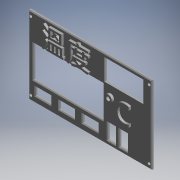
# Autodesk Inventor part: 溫度
Saved by Autodesk Inventor 2021 (Build 250183000, 183)
## iProperties
Part Number: 溫度
Material: 一般
Document SubType Name: 塑型
Designer: aura0
Appearance: 預設
Author: aura0
Autodesk Inventor part; units mm, degrees
ref_plane "YZ 平面" through (0, 0, 0) normal (1, 0, 0) x (0, 1, 0)
ref_plane "XZ 平面" through (0, 0, 0) normal (0, 1, 0) x (-1, 0, 0)
ref_plane "XY 平面" through (0, 0, 0) normal (0, 0, 1) x (1, 0, 0)
sketch "草圖1" plane through (0, 0, 0) normal (0, 0, 1) x (1, 0, 0)
  line L0 (-81, -51) -> (81, -51)
  line L1 (81, -51) -> (81, 51)
  line L2 (81, 51) -> (-81, 51)
  line L3 (-81, 51) -> (-81, -51)
  line L4 (-81, -51) -> (81, 51) construction
  line L5 (81, -51) -> (-81, 51) construction
  point P0 (0, 0)
  dimension "d0" = 162
  dimension "d1" = 102
  constraints: 12 end point, 2 midpoint, 2 parallel, 1 horizontal, 1 perpendicular
  measures "d0" distance of L2.end L1.end
  measures "d1" distance of L1.end L0.end
extrude "擠出1" add sketch "草圖1" along normal blind 3
sketch "草圖2" plane through (0, 0, 3) normal (0, 0, 1) x (1, 0, 0)
  line L0 (-75, -26) -> (17, -26)
  line L1 (17, -26) -> (17, 16)
  line L2 (17, 16) -> (-75, 16)
  line L3 (-75, 16) -> (-75, -26)
  line L4 (19, 19) -> (70, 19)
  line L5 (70, 19) -> (70, 47)
  line L6 (70, 47) -> (19, 47)
  line L7 (19, 47) -> (19, 19)
  line L8 (-72.2, -43) -> (-51.7, -43)
  line L9 (-51.7, -43) -> (-51.7, -32.5)
  line L10 (-51.7, -32.5) -> (-72.2, -32.5)
  line L11 (-72.2, -32.5) -> (-72.2, -43)
  line L12 (-41.2, -43) -> (-20.7, -43)
  line L13 (-20.7, -43) -> (-20.7, -32.5)
  line L14 (-20.7, -32.5) -> (-41.2, -32.5)
  line L15 (-41.2, -32.5) -> (-41.2, -43)
  line L16 (-10.2, -43) -> (10.3, -43)
  line L17 (10.3, -43) -> (10.3, -32.5)
  line L18 (10.3, -32.5) -> (-10.2, -32.5)
  line L19 (-10.2, -32.5) -> (-10.2, -43)
  line L20 (22.8, -45.9) -> (33.3, -45.9)
  line L21 (33.3, -45.9) -> (33.3, -25.4)
  line L22 (33.3, -25.4) -> (22.8, -25.4)
  line L23 (22.8, -25.4) -> (22.8, -45.9)
  line L24 (38.3, -45.9) -> (48.8, -45.9)
  line L25 (48.8, -45.9) -> (48.8, -25.4)
  line L26 (48.8, -25.4) -> (38.3, -25.4)
  line L27 (38.3, -25.4) -> (38.3, -45.9)
  line L28 (-81, -51) -> (81, -51) projected
  line L29 (-81, 51) -> (-81, -51) projected
  point P0 (0, 0)
  dimension "d4" = 8
  dimension "d5" = 8.8
  dimension "d6" = 10.5
  dimension "d7" = 10.5
  dimension "d8" = 10.5
  dimension "d9" = 20.5
  dimension "d10" = 20.5
  dimension "d11" = 20.5
  dimension "d12" = 10.5
  dimension "d13" = 25
  dimension "d14" = 6
  dimension "d15" = 92
  dimension "d16" = 42
  dimension "d17" = 5.1
  dimension "d18" = 10.5
  dimension "d19" = 10.5
  dimension "d20" = 20.5
  dimension "d21" = 5
  dimension "d22" = 103.8
  dimension "d23" = 70
  dimension "d24" = 100
  dimension "d25" = 51
  dimension "d26" = 28
  constraints: 56 end point, 14 parallel, 7 horizontal, 7 perpendicular, 6 point on line
  measures "d4" distance between parallel lines of L28 L8
  measures "d5" distance between parallel lines of L29 L11
  measures "d6" distance between parallel lines of L15 L9
  measures "d7" distance between parallel lines of L19 L13
  measures "d8" distance of L10.end L8.start
  measures "d9" distance of L8.start L8.end
  measures "d10" distance of L16.start L16.end
  measures "d11" distance of L12.start L12.end
  measures "d12" distance of L14.end L12.start
  measures "d13" distance between parallel lines of L28 L0
  measures "d14" distance between parallel lines of L29 L3
  measures "d15" distance of L0.start L0.end
  measures "d16" distance of L2.end L0.start
  measures "d17" distance between parallel lines of L28 L20
  measures "d18" distance of L24.start L24.end
  measures "d19" distance of L20.start L20.end
  measures "d20" distance of L22.end L20.start
  measures "d21" distance between parallel lines of L27 L21
  measures "d22" distance between parallel lines of L29 L23
  measures "d23" distance between parallel lines of L28 L4
  measures "d24" distance between parallel lines of L29 L7
  measures "d25" distance of L4.start L4.end
  measures "d26" distance of L4.end L5.end
extrude "擠出2" cut sketch "草圖2" against normal blind 3
sketch "草圖3" plane through (0, 0, 3) normal (0, 0, 1) x (1, 0, 0)
  line L0 (-63.5264, 47.7672) -> (2.568, 47.7672) construction
  line L1 (2.568, 47.7672) -> (2.568, 18.4539) construction
  line L2 (2.568, 18.4539) -> (-63.5264, 18.4539) construction
  line L3 (-63.5264, 18.4539) -> (-63.5264, 47.7672) construction
  line L4 (20.0661, 9.7884) -> (55.7099, 9.7884) construction
  line L5 (55.7099, 9.7884) -> (55.7099, -16.0486) construction
  line L6 (55.7099, -16.0486) -> (20.0661, -16.0486) construction
  line L7 (20.0661, -16.0486) -> (20.0661, 9.7884) construction
  line L8 (-32.3891, 19.2693) -> (-54.4492, 19.2693)
  line L9 (-54.4492, 19.2693) -> (-54.4492, 21.9303)
  line L10 (-54.4492, 21.9303) -> (-52.5822, 21.9303)
  line L11 (-52.5822, 21.9303) -> (-52.5822, 31.6727)
  line L12 (-52.5822, 31.6727) -> (-33.9771, 31.6727)
  line L13 (-33.9771, 31.6727) -> (-33.9771, 21.9303)
  line L14 (-33.9771, 21.9303) -> (-32.3891, 21.9303)
  line L15 (-32.3891, 21.9303) -> (-32.3891, 19.2693)
  line L16 (-34.6638, 33.7972) -> (-51.9813, 33.7972)
  line L17 (-51.9813, 33.7972) -> (-51.9813, 47.0805)
  line L18 (-51.9813, 47.0805) -> (-34.6638, 47.0805)
  line L19 (-34.6638, 47.0805) -> (-34.6638, 33.7972)
  line L20 (-37.5822, 36.4367) -> (-37.5822, 44.441)
  line L21 (-37.5822, 44.441) -> (-49.0414, 44.441)
  line L22 (-49.0414, 44.441) -> (-49.0414, 36.4367)
  line L23 (-49.0414, 36.4367) -> (-37.5822, 36.4367)
  spline S0 degree 2 poles (-53.7839, 29.2049) (-55.7367, 23.2393) (-58.6122, 18.4539) knots 0 0 0 1 1 1
  line L24 (-58.6122, 18.4539) -> (-61.0371, 20.3852)
  spline S1 degree 2 poles (-61.0371, 20.3852) (-58.2904, 25.0633) (-56.123, 31.029) knots 0 0 0 1 1 1
  line L25 (-56.123, 31.029) -> (-53.7839, 29.2049)
  line L26 (-38.0114, 38.9903) -> (-39.7281, 36.9303)
  spline S2 degree 2 poles (-39.7281, 36.9303) (-41.5092, 38.6255) (-43.505, 39.8058) knots 0 0 0 1 1 1
  spline S3 degree 2 poles (-43.505, 39.8058) (-45.1573, 38.0676) (-46.6809, 37.1878) knots 0 0 0 1 1 1
  line L27 (-46.6809, 37.1878) -> (-48.6122, 39.0547)
  spline S4 degree 2 poles (-48.6122, 39.0547) (-45.2217, 41.0075) (-43.9985, 43.9045) knots 0 0 0 1 1 1
  line L28 (-43.9985, 43.9045) -> (-41.2947, 43.5397)
  spline S5 degree 2 poles (-41.2947, 43.5397) (-41.4449, 42.6813) (-41.9813, 41.8444) knots 0 0 0 1 1 1
  spline S6 degree 2 poles (-41.9813, 41.8444) (-39.4921, 40.3423) (-38.0114, 38.9903) knots 0 0 0 1 1 1
  line L29 (-52.7539, 42.9388) -> (-54.8354, 40.6642)
  spline S7 degree 2 poles (-54.8354, 40.6642) (-56.7238, 42.8745) (-60.565, 45.4925) knots 0 0 0 1 1 1
  line L30 (-60.565, 45.4925) -> (-58.4835, 47.7028)
  spline S8 degree 2 poles (-58.4835, 47.7028) (-54.9427, 45.4066) (-52.7539, 42.9388) knots 0 0 0 1 1 1
  line L31 (-53.6552, 34.9775) -> (-55.5221, 32.6813)
  spline S9 degree 2 poles (-55.5221, 32.6813) (-57.7968, 35.0204) (-61.4663, 37.3594) knots 0 0 0 1 1 1
  line L32 (-61.4663, 37.3594) -> (-59.5994, 39.6985)
  spline S10 degree 2 poles (-59.5994, 39.6985) (-55.8226, 37.3165) (-53.6552, 34.9775) knots 0 0 0 1 1 1
  line L33 (-36.6595, 21.9303) -> (-36.6595, 29.0333)
  line L34 (-36.6595, 29.0333) -> (-39.2775, 29.0333)
  line L35 (-39.2775, 29.0333) -> (-39.2775, 21.9303)
  line L36 (-39.2775, 21.9303) -> (-36.6595, 21.9303)
  line L37 (-42.0243, 21.9303) -> (-42.0243, 29.0333)
  line L38 (-42.0243, 29.0333) -> (-44.5565, 29.0333)
  line L39 (-44.5565, 29.0333) -> (-44.5565, 21.9303)
  line L40 (-44.5565, 21.9303) -> (-42.0243, 21.9303)
  line L41 (-47.2603, 21.9303) -> (-47.2603, 29.0333)
  line L42 (-47.2603, 29.0333) -> (-49.771, 29.0333)
  line L43 (-49.771, 29.0333) -> (-49.771, 21.9303)
  line L44 (-49.771, 21.9303) -> (-47.2603, 21.9303)
  line L45 (0.744, 21.4367) -> (-0.1359, 18.6255)
  spline S11 degree 2 poles (-0.1359, 18.6255) (-6.0586, 18.9689) (-11.2732, 21.0933) knots 0 0 0 1 1 1
  spline S12 degree 2 poles (-11.2732, 21.0933) (-15.5436, 19.3122) (-21.4019, 18.5612) knots 0 0 0 1 1 1
  line L46 (-21.4019, 18.5612) -> (-22.7539, 21.3509)
  spline S13 degree 2 poles (-22.7539, 21.3509) (-17.6895, 21.6298) (-14.4921, 22.853) knots 0 0 0 1 1 1
  spline S14 degree 2 poles (-14.4921, 22.853) (-17.3676, 24.6556) (-18.9127, 27.7457) knots 0 0 0 1 1 1
  line L47 (-18.9127, 27.7457) -> (-20.3719, 27.7457)
  line L48 (-20.3719, 27.7457) -> (-20.3719, 30.3637)
  line L49 (-20.3719, 30.3637) -> (-3.0114, 30.3637)
  line L50 (-3.0114, 30.3637) -> (-3.0114, 27.7457)
  spline S15 degree 2 poles (-3.0114, 27.7457) (-4.7281, 25.1062) (-8.1401, 22.853) knots 0 0 0 1 1 1
  spline S16 degree 2 poles (-8.1401, 22.853) (-4.3848, 21.544) (0.744, 21.4367) knots 0 0 0 1 1 1
  line L51 (0.5508, 42.7457) -> (-22.4749, 42.7457)
  line L52 (-22.4749, 42.7457) -> (-22.4749, 31.9088)
  spline S17 degree 2 poles (-22.4749, 31.9088) (-22.4749, 23.7972) (-25.8869, 18.5612) knots 0 0 0 1 1 1
  line L53 (-25.8869, 18.5612) -> (-28.3547, 20.2135)
  spline S18 degree 2 poles (-28.3547, 20.2135) (-25.4363, 24.677) (-25.4363, 31.9088) knots 0 0 0 1 1 1
  line L54 (-25.4363, 31.9088) -> (-25.4363, 45.3637)
  line L55 (-25.4363, 45.3637) -> (-14.5779, 45.3637)
  spline S19 degree 2 poles (-14.5779, 45.3637) (-15.2217, 46.3509) (-15.844, 47.0805) knots 0 0 0 1 1 1
  line L56 (-15.844, 47.0805) -> (-12.6251, 47.7672)
  spline S20 degree 2 poles (-12.6251, 47.7672) (-11.9813, 46.6727) (-11.2517, 45.3637) knots 0 0 0 1 1 1
  line L57 (-11.2517, 45.3637) -> (0.5508, 45.3637)
  line L58 (0.5508, 45.3637) -> (0.5508, 42.7457)
  line L59 (0.229, 37.1019) -> (-4.6208, 37.1019)
  line L60 (-4.6208, 37.1019) -> (-4.6208, 32.2307)
  line L61 (-4.6208, 32.2307) -> (-17.3891, 32.2307)
  line L62 (-17.3891, 32.2307) -> (-17.3891, 37.1019)
  line L63 (-17.3891, 37.1019) -> (-21.359, 37.1019)
  line L64 (-21.359, 37.1019) -> (-21.359, 39.677)
  line L65 (-21.359, 39.677) -> (-17.3891, 39.677)
  line L66 (-17.3891, 39.677) -> (-17.3891, 41.6298)
  line L67 (-17.3891, 41.6298) -> (-14.5565, 41.6298)
  line L68 (-14.5565, 41.6298) -> (-14.5565, 39.677)
  line L69 (-14.5565, 39.677) -> (-7.5178, 39.677)
  line L70 (-7.5178, 39.677) -> (-7.5178, 41.6298)
  line L71 (-7.5178, 41.6298) -> (-4.6208, 41.6298)
  line L72 (-4.6208, 41.6298) -> (-4.6208, 39.677)
  line L73 (-4.6208, 39.677) -> (0.229, 39.677)
  line L74 (0.229, 39.677) -> (0.229, 37.1019)
  line L75 (-6.7668, 27.7457) -> (-15.5007, 27.7457)
  spline S21 degree 2 poles (-15.5007, 27.7457) (-14.1702, 25.7071) (-11.4019, 24.0976) knots 0 0 0 1 1 1
  spline S22 degree 2 poles (-11.4019, 24.0976) (-8.2689, 25.9002) (-6.7668, 27.7457) knots 0 0 0 1 1 1
  line L76 (-7.5178, 34.7843) -> (-7.5178, 37.1019)
  line L77 (-7.5178, 37.1019) -> (-14.5565, 37.1019)
  line L78 (-14.5565, 37.1019) -> (-14.5565, 34.7843)
  line L79 (-14.5565, 34.7843) -> (-7.5178, 34.7843)
  spline S23 degree 2 poles (26.8687, 9.7884) (28.8859, 9.7884) (31.7399, 6.9343) (31.7399, 4.96) knots 0 0 0 1 2 2 2
  spline S24 degree 2 poles (31.7399, 4.96) (31.7399, 2.9643) (28.8644, 0.0888) (26.8687, 0.0888) knots 0 0 0 1 2 2 2
  spline S25 degree 2 poles (26.8687, 0.0888) (24.8515, 0.0888) (21.9975, 2.9643) (21.9975, 4.96) knots 0 0 0 1 2 2 2
  spline S26 degree 2 poles (21.9975, 4.96) (21.9975, 6.9343) (24.873, 9.7884) (26.8687, 9.7884) knots 0 0 0 1 2 2 2
  spline S27 degree 2 poles (26.8687, 2.3635) (27.9417, 2.3635) (29.4438, 3.9085) (29.4438, 4.96) knots 0 0 0 1 2 2 2
  spline S28 degree 2 poles (29.4438, 4.96) (29.4438, 6.0115) (27.9417, 7.5137) (26.8687, 7.5137) knots 0 0 0 1 2 2 2
  spline S29 degree 2 poles (26.8687, 7.5137) (25.8172, 7.5137) (24.3151, 6.0115) (24.3151, 4.96) knots 0 0 0 1 2 2 2
  spline S30 degree 2 poles (24.3151, 4.96) (24.3151, 3.9085) (25.8172, 2.3635) (26.8687, 2.3635) knots 0 0 0 1 2 2 2
  spline S31 degree 2 poles (54.0146, -14.6322) (51.2464, -16.0486) (47.0404, -16.0486) knots 0 0 0 1 1 1
  spline S32 degree 2 poles (47.0404, -16.0486) (41.6112, -16.0486) (35.0876, -9.2031) (35.0876, -3.6237) knots 0 0 0 1 2 2 2
  spline S33 degree 2 poles (35.0876, -3.6237) (35.0876, 2.2347) (42.3193, 9.7884) (48.049, 9.7884) knots 0 0 0 1 2 2 2
  spline S34 degree 2 poles (48.049, 9.7884) (51.6326, 9.7884) (54.0146, 8.8012) knots 0 0 0 1 1 1
  line L80 (54.0146, 8.8012) -> (54.0146, 4.8742)
  spline S35 degree 2 poles (54.0146, 4.8742) (51.3751, 6.3549) (48.1777, 6.3549) knots 0 0 0 1 1 1
  spline S36 degree 2 poles (48.1777, 6.3549) (44.079, 6.3549) (39.1434, 0.9901) (39.1434, -3.3662) knots 0 0 0 1 2 2 2
  spline S37 degree 2 poles (39.1434, -3.3662) (39.1434, -7.5078) (43.7786, -12.6365) (47.6627, -12.6365) knots 0 0 0 1 2 2 2
  spline S38 degree 2 poles (47.6627, -12.6365) (51.2893, -12.6365) (54.0146, -10.9627) knots 0 0 0 1 1 1
  line L81 (54.0146, -10.9627) -> (54.0146, -14.6322)
  point P0 (0, 0)
  constraints: 4 other
extrude "擠出3" add sketch "草圖3" along normal blind 3
sketch "草圖4" plane through (0, 0, 3) normal (0, 0, 1) x (1, 0, 0)
  circle A0 centre (-77.9, 45) radius 1.8
  circle A1 centre (-77.9, -45) radius 1.8
  circle A2 centre (77.7, -45) radius 1.8
  circle A3 centre (77.7, 45) radius 1.8
  line L0 (-81, -51) -> (81, -51) projected
  line L1 (-81, 51) -> (-81, -51) projected
  point P0 (0, 0)
  dimension "d31" = 6
  dimension "d32" = 3.1
  dimension "d33" = 3.1
  dimension "d34" = 6
  dimension "d35" = 158.7
  dimension "d36" = 96
  dimension "d37" = 96
  dimension "d38" = 158.7
  dimension "d39" = 3.6
  dimension "d40" = 3.6
  dimension "d41" = 3.6
  dimension "d42" = 3.6
  constraints: 4 centre point
  measures "d31" distance from line of L0 A1.centre
  measures "d32" distance from line of L1 A1.centre
  measures "d33" distance from line of L1 A0.centre
  measures "d34" distance from line of L0 A2.centre
  measures "d35" distance from line of L1 A2.centre
  measures "d36" distance from line of L0 A0.centre
  measures "d37" distance from line of L0 A3.centre
  measures "d38" distance from line of L1 A3.centre
  measures "d39" diameter of A1
  measures "d40" diameter of A0
  measures "d41" diameter of A3
  measures "d42" diameter of A2
extrude "擠出4" cut sketch "草圖4" against normal blind 3
chamfer "倒角1" distance 1 angle 45 28 edges at (-29, 16, 3) (-29, -26, 3) (17, -5, 3) (-75, -5, 3) (-81, 0, 3) (0, 51, 3) (81, 0, 3) (0, -51, 3) (33.3, -35.65, 3) (28.05, -25.4, 3) (22.8, -35.65, 3) (28.05, -45.9, 3) (38.3, -35.65, 3) (43.55, -25.4, 3) (48.8, -35.65, 3) (43.55, -45.9, 3) (0.05, -43, 3) (10.3, -37.75, 3) (0.05, -32.5, 3) (-10.2, -37.75, 3) (-20.7, -37.75, 3) (-30.95, -32.5, 3) (-30.95, -43, 3) (-41.2, -37.75, 3) (-51.7, -37.75, 3) (-61.95, -32.5, 3) (-61.95, -43, 3) (-72.2, -37.75, 3)
equation "\"d7\" = d6"
equation "\"d10\" = d9"
equation "\"d11\" = d9"
equation "\"d18\" = d12"
equation "\"d19\" = d12"
equation "\"d20\" = d10"
equation "\"d33\" = d32"
equation "\"d34\" = d31"
equation "\"d37\" = d36"
equation "\"d38\" = d35"
equation "\"d40\" = d39"
equation "\"d41\" = d39"
equation "\"d42\" = d39"
